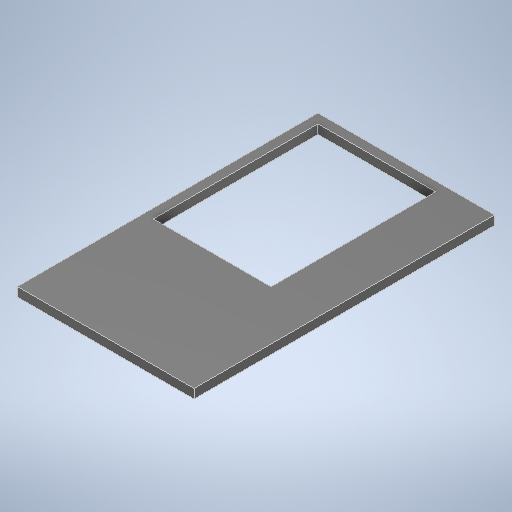
# Autodesk Inventor part: lid
Saved by Autodesk Inventor 2025.2 (Build 292293000, 293)
## iProperties
Created: 2025-08-16
Part Number: lid
Material: Acetal Resin, Black
Document SubType Name: Modeling
Designer: pakiyan
Density: 1.425 g/cm^3
Appearance: Smooth - Black
Author: pakiyan
Autodesk Inventor part; units mm, degrees
ref_plane "YZ Plane" through (0, 0, 0) normal (1, 0, 0) x (0, 1, 0)
ref_plane "XZ Plane" through (0, 0, 0) normal (0, 1, 0) x (-1, 0, 0)
ref_plane "XY Plane" through (0, 0, 0) normal (0, 0, 1) x (1, 0, 0)
sketch "Sketch1" plane through (0, 0, 0) normal (0, 1, 0) x (-1, 0, 0)
  line L0 (37.6, 64) -> (-37.6, 64)
  line L1 (-37.6, 64) -> (-37.6, -64)
  line L2 (-37.6, -64) -> (37.6, -64)
  line L3 (37.6, -64) -> (37.6, 64)
  line L4 (37.6, 64) -> (-37.6, -64) construction
  line L5 (-37.6, 64) -> (37.6, -64) construction
  line L6 (33.6, 10.1) -> (-16.5, 10.1)
  line L7 (-16.5, 10.1) -> (-16.5, -60)
  line L8 (-16.5, -60) -> (33.6, -60)
  line L9 (33.6, -60) -> (33.6, 10.1)
  line L10 (33.6, 10.1) -> (-16.5, -60) construction
  line L11 (-16.5, 10.1) -> (33.6, -60) construction
  point P0 (0, 0)
  dimension "d0" = 128
  dimension "d1" = 75.2
  dimension "d2" = 70.1
  dimension "d3" = 50.1
  dimension "d4" = 4
  dimension "d5" = 4
  constraints: 24 end point, 4 parallel, 2 horizontal, 2 midpoint, 2 perpendicular
  measures "d0" distance of L0.end L1.end
  measures "d1" distance of L1.end L2.end
  measures "d2" distance of L6.end L7.end
  measures "d3" distance of L7.end L8.end
  measures "d4" distance between parallel lines of L3 L9
  measures "d5" distance between parallel lines of L2 L8
extrude "Extrusion1" add sketch "Sketch1" along normal blind 3.9
body "Solid1"
